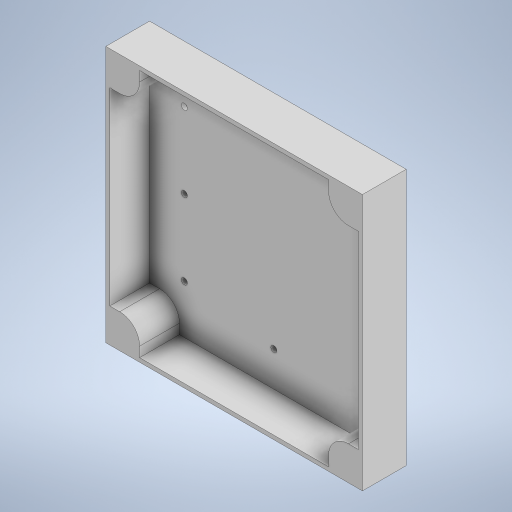
# Autodesk Inventor part: Gehäuse_Sensor_Dummy
Saved by Autodesk Inventor 2023 (Build 270158000, 158)
## iProperties
Created: 2022-12-01
Part Number: Gehäuse_Sensor_Dummy
Material: Generisch
Document SubType Name: Modeling
Designer: Admin
Density: 1 g/cm^3
Appearance: Vorgabe
Author: Admin
Autodesk Inventor part; units mm, degrees
ref_plane "YZ Plane" through (0, 0, 0) normal (1, 0, 0) x (0, 1, 0)
ref_plane "XZ Plane" through (0, 0, 0) normal (0, 1, 0) x (-1, 0, 0)
ref_plane "XY Plane" through (0, 0, 0) normal (0, 0, 1) x (1, 0, 0)
sketch "Skizze1" plane through (0, 0, 0) normal (0, 0, 1) x (1, 0, 0)
  line L0 (-64.5, 64.5) -> (64.5, 64.5)
  line L1 (64.5, 64.5) -> (64.5, -64.5)
  line L2 (64.5, -64.5) -> (-64.5, -64.5)
  line L3 (-64.5, -64.5) -> (-64.5, 64.5)
  line L4 (-64.5, 64.5) -> (64.5, -64.5) construction
  line L5 (64.5, 64.5) -> (-64.5, -64.5) construction
  point P0 (0, 0)
  dimension "d0" = 129
  dimension "d1" = 129
  constraints: 12 end point, 2 midpoint, 2 parallel, 1 horizontal, 1 perpendicular
  measures "d0" distance of L0.start L0.end
  measures "d1" distance of L0.end L1.end
extrude "Extrusion1" add sketch "Skizze1" along normal blind 2
sketch "Skizze2" plane through (0, 0, 2) normal (0, 0, 1) x (1, 0, 0)
  line L0 (64.5, 64.5) -> (-64.5, 64.5) projected
  line L1 (-64.5, -64.5) -> (64.5, -64.5) projected
  line L2 (-64.5, 64.5) -> (64.5, 64.5)
  line L3 (64.5, 64.5) -> (64.5, -64.5)
  line L4 (64.5, -64.5) -> (-64.5, -64.5)
  line L5 (-64.5, -64.5) -> (-64.5, 64.5)
  line L6 (62.5, -47.5) -> (62.5, 47.5)
  line L7 (47.5, 62.5) -> (-47.5, 62.5)
  line L8 (-62.5, 47.5) -> (-62.5, -47.5)
  line L9 (-47.5, -62.5) -> (47.5, -62.5)
  line L10 (-47.5, 62.5) -> (-47.5, 57.5)
  line L11 (-57.5, 47.5) -> (-62.5, 47.5)
  line L12 (47.5, 62.5) -> (47.5, 57.5)
  line L13 (57.5, 47.5) -> (62.5, 47.5)
  line L14 (62.5, -47.5) -> (57.5, -47.5)
  line L15 (47.5, -57.5) -> (47.5, -62.5)
  line L16 (-62.5, -47.5) -> (-57.5, -47.5)
  line L17 (-47.5, -57.5) -> (-47.5, -62.5)
  arc A0 (-57.5, 47.5) -> (-47.5, 57.5) centre (-57.5, 57.5) ccw
  arc A1 (47.5, 57.5) -> (57.5, 47.5) centre (57.5, 57.5) ccw
  arc A2 (57.5, -47.5) -> (47.5, -57.5) centre (57.5, -57.5) ccw
  arc A3 (-47.5, -57.5) -> (-57.5, -47.5) centre (-57.5, -57.5) ccw
  point P0 (0, 0)
  point P1 (47.5, 47.5)
  point P2 (47.5, -47.5)
  point P3 (-47.5, -47.5)
  dimension "d4" = 2
  dimension "d5" = 17
  dimension "d8" = 10
  dimension "d9" = 2
  dimension "d10" = 2
  dimension "d11" = 2
  constraints: 32 end point, 12 point on line, 9 perpendicular, 8 point on circle, 8 tangent, 5 parallel, 4 centre point, 3 equal radius, 1 horizontal, 1 vertical
  measures "d4" distance between parallel lines of L3 L6
  measures "d5" distance between parallel lines of L5 L10
  measures "d8" radius of A0
  measures "d9" distance between parallel lines of L0 L7
  measures "d10" distance between parallel lines of L5 L8
  measures "d11" distance between parallel lines of L9 L4
extrude "Extrusion2" add sketch "Skizze2" along normal blind 20
sketch "Skizze3" plane through (0, 0, 2) normal (0, 0, 1) x (1, 0, 0)
  line L0 (-45, 38) -> (45, 38)
  line L1 (45, 38) -> (45, -38)
  line L2 (45, -38) -> (-45, -38)
  line L3 (-45, -38) -> (-45, 38)
  line L4 (-45, 38) -> (45, -38) construction
  line L5 (45, 38) -> (-45, -38) construction
  line L6 (64.5, 64.5) -> (-64.5, 64.5) projected
  line L7 (0, 64.5) -> (0, 45)
  line L8 (0, -45) -> (0, -64.5)
  line L9 (-64.5, -64.5) -> (64.5, -64.5) projected
  point P0 (0, 0)
  point P1 (45, 0)
  point P2 (-45, 0)
  dimension "d14" = 76
  dimension "d15" = 90
  dimension "d16" = 90
  constraints: 16 end point, 6 midpoint, 5 coincident, 2 parallel, 2 vertical, 1 collinear, 1 horizontal, 1 perpendicular
  measures "d14" distance of L2.end L0.start
  measures "d15" distance of L1.end L2.end
  measures "d16" distance of L8.start point (0, 45)
hole "Bohrung1" at (-45, 38, 2) at (45, 38, 2) at (45, 0, 2) at (45, -38, 2) at (-45, -38, 2) at (-45, 0, 2) at (0, 45, 2) at (0, -45, 2) direction (0, 0, -1) diameter 3 end through all
